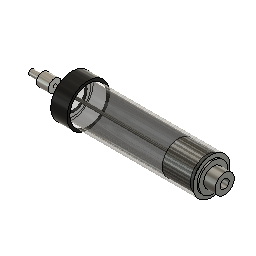
Inkwell_v0.2 (Autodesk Fusion 360 archive; units mm, degrees)
design "Dashpot"
Autodesk Fusion 360 part; units mm, degrees
sketch "Sketch1" plane through (0, 0, 0) normal (0, 0, 1) x (1, 0, 0)
  line L0 (8.1, 9.19) -> (69.35, 9.19)
  line L1 (8.1, 9.19) -> (8.1, 10.5156)
  line L2 (8.1, 10.5156) -> (0, 10.5156)
  line L3 (0, 10.5156) -> (0, 6.5)
  line L4 (1, 8.19) -> (68.35, 8.19)
  line L5 (68.35, 8.19) -> (68.35, 2.2)
  line L6 (68.35, 2.2) -> (75.9, 2.2)
  line L7 (75.9, 2.2) -> (75.9, 4.7625)
  line L8 (75.9, 4.7625) -> (70.2, 4.7625)
  line L9 (70.2, 4.7625) -> (70.2, 7.19)
  line L10 (0, 6.5) -> (1, 6.5)
  line L11 (1, 6.5) -> (1, 8.19)
  line L12 (69.35, 9.19) -> (69.35, 7.19)
  line L13 (69.35, 7.19) -> (70.2, 7.19)
  line L14 (0, 0) -> (87.0356, 0) construction
  line L15 (67.08, 0) -> (63.08, 0)
  line L16 (53.07, 6.19) -> (53.07, 8.19)
  line L17 (53.07, 8.19) -> (67.08, 8.19)
  line L18 (67.08, 8.19) -> (67.08, 0)
  line L19 (63.08, 0) -> (63.08, 6.19)
  line L20 (63.08, 6.19) -> (53.07, 6.19)
  line L21 (63.08, 0) -> (-20.2, 0)
  line L22 (-20.2, 0) -> (-20.2, 1.4224)
  line L23 (-20.2, 1.4224) -> (-14.5, 1.4224)
  line L24 (-14.5, 1.4224) -> (-14.5, 3.2)
  line L25 (-14.5, 3.2) -> (-8.6, 3.2)
  line L26 (-8.6, 3.2) -> (-8.6, 0.715)
  line L27 (-8.6, 0.715) -> (63.08, 0.715)
  dimension "d2" = 1
  dimension "d3" = 0.85
  dimension "d5" = 1
  dimension "d6" = 9.19
  dimension "d7" = 10.5156
  dimension "d8" = 8.1
  dimension "d9" = 6.5
  dimension "d10" = 2
  dimension "d11" = 1
  dimension "d12" = 4.7625
  dimension "d13" = 2.2
  dimension "d14" = 5.7
  dimension "d15" = 70.2
  dimension "d16" = 1.27
  dimension "d17" = 52.07
  dimension "d18" = 2
  dimension "d19" = 4
  dimension "d20" = 0.715
  dimension "d21" = 8.6
  dimension "d22" = 1.4224
  dimension "d23" = 5.9
  dimension "d24" = 3.2
  dimension "d25" = 5.7
  constraint horizontal L0
  constraint perpendicular L0 L1
  constraint perpendicular L1 L2
  constraint perpendicular L2 L3
  constraint perpendicular L3 L4
  constraint perpendicular L4 L5
  constraint perpendicular L5 L6
  constraint perpendicular L6 L7
  constraint perpendicular L5 L8
  constraint perpendicular L3 L10
  constraint vertical L11
  constraint vertical L9
  constraint perpendicular L0 L12
  constraint horizontal L13
  constraint coincident L14.start origin
  constraint horizontal L14
  constraint coincident L14.start L3
  constraint horizontal L15
  constraint vertical L16
  constraint horizontal L17
  constraint vertical L18
  constraint coincident L14 L15.start
  constraint perpendicular L15 L19
  constraint horizontal L20
  constraint perpendicular L19 L21
  constraint perpendicular L21 L22
  constraint perpendicular L22 L23
  constraint perpendicular L21 L24
  constraint perpendicular L22 L25
  constraint perpendicular L21 L26
  constraint coincident L19 L27.end
  constraint perpendicular L19 L27
  constraint coincident L4 L16.end
  measures "d2" distance of L0 L4
  measures "d3" distance of L9.end L12.end
  measures "d5" distance of L3.end L10.end
  measures "d6" distance of L0 L14
  measures "d7" distance of L2 L14
  measures "d8" distance of L1.end L2.end
  measures "d9" distance of L14.start L10
  measures "d10" distance of L0.end L12.end
  measures "d11" distance of L5 L12
  measures "d12" distance of L8 L14
  measures "d13" distance of L6 L14
  measures "d14" distance of L7.end L8.end
  measures "d15" distance of L3 L9
  measures "d16" distance of L5 L18
  measures "d17" distance of L11 L16
  measures "d18" distance of L16.start L16.end
  measures "d19" distance of L18 L19
  measures "d20" distance of L21 L27
  measures "d21" distance of L3 L26
  measures "d22" distance of L21 L23
  measures "d23" distance of L24.end L25.end
  measures "d24" distance of L21 L25
  measures "d25" distance of L22.end L23.end
revolve "Revolve1" add sketch "Sketch1" angle 360 about axis through (0, 0, 0) along (1, 0, 0) contours L0 L1 L2 L3 L4 L5 L6 L7 L8 L9 L10 L11 L12 L13 L17 makes body 1
revolve "Revolve2" add sketch "Sketch1" angle 360 about axis through (0, 0, 0) along (1, 0, 0) separate body contours L4 L15 L16 L17 L18 L19 L20 | L19 L21 L22 L23 L24 L25 L26 L27 makes body 2
copy_body "Body->Comp1" bodies 1 removing the originals makes body 3 in component "DashpotBody"
copy_body "Body->Comp2" bodies 2 removing the originals makes body 4 in component "DashpotPlunger"
component "DashpotBody" placed x (1, 0, 0) y (0, 1, 0) z (0, 0, 1) at (0, 0, 0)
component "DashpotPlunger" placed x (1, 0, 0) y (0, 1, 0) z (0, 0, 1) at (0, 0, 0)
equation "d6 = 18.38 mm / 2"
equation "d7 = 0.828 in / 2"
equation "d9 = ( 13 / 2 ) * 1 mm"
equation "d12 = 3 / 8 / 2 * 1 in"
equation "d13 = 4.4 mm / 2"
equation "d20 = ( 1.43 / 2 ) * 1 mm"
equation "d22 = ( 0.112 / 2 ) * 1 in"
equation "d24 = ( 6.4 / 2 ) * 1 mm"

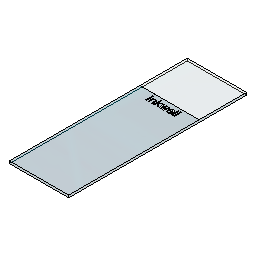
design "Slide"
Autodesk Fusion 360 part; units mm, degrees
sketch "Sketch1" plane through (0, 0, 0) normal (0, 1, 0) x (1, 0, 0)
  line L0 (-12.5, 37.5) -> (12.5, 37.5)
  line L1 (12.5, 37.5) -> (12.5, -37.5)
  line L2 (12.5, -37.5) -> (-12.5, -37.5)
  line L3 (-12.5, -37.5) -> (-12.5, 37.5)
  line L4 (-12.5, 37.5) -> (12.5, -37.5) construction
  dimension "d1" = 25
  dimension "d2" = 75
  constraint horizontal L0
  constraint vertical L1
  constraint horizontal L2
  constraint vertical L3
  constraint midpoint origin L4
  measures "d1" distance of L0.start L0.end
  measures "d2" distance of L0.start L2.end
extrude "Extrude1" add sketch "Sketch1" along normal blind 1
sketch "Sketch2" plane through (0, 1, 0) normal (0, 1, 0) x (-1, 0, 0)
  line L0 (12.5, 37.5) -> (-12.5, 37.5)
  line L1 (-12.5, 37.5) -> (-12.5, -37.5)
  line L2 (-12.5, -37.5) -> (12.5, -37.5)
  line L3 (12.5, -37.5) -> (12.5, 37.5)
  line L4 (12.5, -17.5) -> (-12.5, -17.5)
  line L5 (7.5, -13.5) -> (-7.5, -13.5) construction
  line L6 (-7.5, -13.5) -> (-7.5, -17.5) construction
  line L7 (-7.5, -17.5) -> (7.5, -17.5) construction
  line L8 (7.5, -17.5) -> (7.5, -13.5) construction
  dimension "d5" = 20
  dimension "d8" = 3
  dimension "d9" = 24
  dimension "d10" = 15
  text T0 "Inkwell" font "Arial" height 3 align centre bottom in box 15 x 4 at (7.5, -13.5) x (-1, 0) y (0, -1) spacing 1 kerned
  constraint coincident L3 L4.start
  constraint coincident L1 L4.end
  constraint perpendicular L1 L4
  constraint vertical origin
  constraint coincident L4
  measures "d5" distance of L2 L4
  measures "d9" distance of L2 L5
extrude "Extrude2" add sketch "Sketch2" sketch "Sketch2" along normal blind 0.01 contours L1 L2 L3 L4 of sketch 2 text T0
